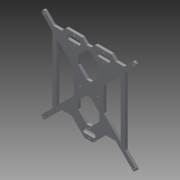
# Autodesk Inventor part: platform_redrawn
Saved by Autodesk Inventor 2015 (Build 190159000, 159)
## iProperties
Created: 2015-04-29
Part Number: platform_redrawn
Material: Generic
Document SubType Name: Modeling
Designer: X
Density: 1 g/cm^3
Appearance: Default
Author: X
Autodesk Inventor part; units mm, degrees
ref_plane "YZ Plane" through (0, 0, 0) normal (1, 0, 0) x (0, 1, 0)
ref_plane "XZ Plane" through (0, 0, 0) normal (0, 1, 0) x (-1, 0, 0)
ref_plane "XY Plane" through (0, 0, 0) normal (0, 0, 1) x (1, 0, 0)
sketch "Sketch1" plane through (0, 0, 0) normal (0, 1, 0) x (-1, 0, 0)
  line L0 (110, 110) -> (-110, 110)
  line L1 (-110, 110) -> (-110, -110)
  line L2 (-110, -110) -> (110, -110)
  line L3 (110, -110) -> (110, 110)
  line L4 (110, 110) -> (-110, -110) construction
  line L5 (-110, 110) -> (110, -110) construction
  point P0 (0, 0)
  dimension "d0" = 220
  dimension "d1" = 220
  constraints: 12 end point, 2 midpoint, 2 parallel, 1 horizontal, 1 perpendicular
  measures "d0" distance of L2.end L0.start
  measures "d1" distance of L0.start L0.end
extrude "Extrusion1" add sketch "Sketch1" along normal blind 6
sketch "Sketch2" plane through (0, 6, 0) normal (0, 1, 0) x (1, 0, 0)
  line L0 (110, 110) -> (-110, 110) construction
  line L1 (0, 110) -> (0, -110) construction
  line L2 (-110, 110) -> (-110, -110) projected
  line L3 (-110, 103) -> (-110, -103)
  line L4 (-110, -103) -> (-85, -78)
  line L5 (-85, -78) -> (-85, 78)
  line L6 (-85, 78) -> (-110, 103)
  line L7 (-75, 68) -> (-75, -68)
  line L8 (-75, -68) -> (-35, -28)
  line L9 (-35, -28) -> (-35, 28)
  line L10 (-35, 28) -> (-75, 68)
  line L11 (-110, -110) -> (110, -110) projected
  line L12 (-103, -110) -> (-83, -90)
  line L13 (-83, -90) -> (-63, -90)
  line L14 (-63, -90) -> (-43, -110)
  line L15 (-103, -110) -> (-43, -110)
  line L16 (-53, -100) -> (-15, -100)
  line L17 (-15, -100) -> (-15, -110)
  line L18 (-15, -110) -> (-53, -110)
  line L19 (-53, -110) -> (-53, -100)
  line L20 (-25, -110) -> (-5, -90)
  line L21 (-5, -90) -> (0, -90)
  line L22 (0, -80) -> (-5, -80)
  line L23 (-5, -80) -> (-25, -60)
  line L24 (-25, -60) -> (-25, -40)
  line L25 (-25, -40) -> (-5, -20)
  line L26 (-5, -20) -> (0, -20)
  line L27 (-103, 110) -> (-63, 70)
  line L28 (-63, 70) -> (-40, 70)
  line L29 (-40, 70) -> (0, 110)
  line L30 (0, 110) -> (-103, 110)
  line L31 (-10, 100) -> (0, 100)
  line L32 (0, 100) -> (0, 110)
  line L33 (0, 110) -> (-10, 110)
  line L34 (-10, 110) -> (-10, 100)
  line L35 (0, 70) -> (-5, 70)
  line L36 (-5, 70) -> (-25, 50)
  line L37 (-25, 50) -> (-25, 32)
  line L38 (-25, 32) -> (-5, 12)
  line L39 (-5, 12) -> (0, 12)
  line L40 (-110, 110) -> (110, 110) construction
  line L41 (110, 110) -> (110, -110)
  line L42 (110, 103) -> (110, -103)
  line L43 (110, -103) -> (85, -78)
  line L44 (85, -78) -> (85, 78)
  line L45 (85, 78) -> (110, 103)
  line L46 (75, 68) -> (75, -68)
  line L47 (75, -68) -> (35, -28)
  line L48 (35, -28) -> (35, 28)
  line L49 (35, 28) -> (75, 68)
  line L50 (110, -110) -> (-110, -110)
  line L51 (103, -110) -> (83, -90)
  line L52 (83, -90) -> (63, -90)
  line L53 (63, -90) -> (43, -110)
  line L54 (103, -110) -> (43, -110)
  line L55 (53, -100) -> (15, -100)
  line L56 (15, -100) -> (15, -110)
  line L57 (15, -110) -> (53, -110)
  line L58 (53, -110) -> (53, -100)
  line L59 (25, -110) -> (5, -90)
  line L60 (5, -90) -> (0, -90)
  line L61 (0, -80) -> (5, -80)
  line L62 (5, -80) -> (25, -60)
  line L63 (25, -60) -> (25, -40)
  line L64 (25, -40) -> (5, -20)
  line L65 (5, -20) -> (0, -20)
  line L66 (103, 110) -> (63, 70)
  line L67 (63, 70) -> (40, 70)
  line L68 (40, 70) -> (0, 110)
  line L69 (0, 110) -> (103, 110)
  line L70 (10, 100) -> (0, 100)
  line L71 (0, 110) -> (10, 110)
  line L72 (10, 110) -> (10, 100)
  line L73 (0, 70) -> (5, 70)
  line L74 (5, 70) -> (25, 50)
  line L75 (25, 50) -> (25, 32)
  line L76 (25, 32) -> (5, 12)
  line L77 (5, 12) -> (0, 12)
  line L78 (-15, -110) -> (0, -110)
  line L79 (110, -110) -> (-110, -110)
  line L80 (-110, -110) -> (110, -110)
  line L81 (15, -110) -> (0, -110)
  point P0 (0, 0)
  dimension "d4" = 206
  dimension "d6" = 25
  dimension "d7" = 135
  dimension "d8" = 7
  dimension "d10" = 10
  dimension "d11" = 40
  dimension "d12" = 135
  dimension "d13" = 7
  dimension "d14" = 20
  dimension "d15" = 135
  dimension "d16" = 38
  dimension "d17" = 10
  dimension "d20" = 25
  dimension "d21" = 60
  dimension "d22" = 10
  dimension "d23" = 135
  dimension "d24" = 57
  dimension "d25" = 7
  dimension "d26" = 40
  dimension "d27" = 10
  dimension "d28" = 30
  constraints: 158 end point, 39 symmetric about line, 21 point on line, 12 parallel, 7 collinear, 7 equal length, 7 perpendicular, 6 midpoint, 5 horizontal, 2 vertical
  measures "d4" distance of L3.end L3.start
  measures "d6" distance between parallel lines of L5 L3
  measures "d7" angle of L5 L6
  measures "d8" distance from line of L0 L3.start
  measures "d10" distance between parallel lines of L7 L5
  measures "d11" distance between parallel lines of L7 L9
  measures "d12" angle of L5 L4
  measures "d13" distance from line of L12.start L2
  measures "d14" distance between parallel lines of L11 L13
  measures "d15" angle of L14 L13
  measures "d16" distance of L16.start L16.end
  measures "d17" distance between parallel lines of L16 L13
  measures "d20" distance between parallel lines of L1 L24
  measures "d21" distance between parallel lines of L22 L26
  measures "d22" distance between parallel lines of L21 L22
  measures "d23" angle of L23 L24
  measures "d24" distance between parallel lines of L2 L19
  measures "d25" distance from line of L2 L27.start
  measures "d26" distance between parallel lines of L0 L28
  measures "d27" distance between parallel lines of L0 L31
  measures "d28" distance between parallel lines of L35 L31
extrude "Extrusion2" cut sketch "Sketch2" against normal through all
chamfer "Chamfer3" distance 3 angle 45 1 edges at (-110, 3, 110) measured on face at (-109.5, 3, 110)
chamfer "Chamfer4" distance 3 angle 45 1 edges at (110, 3, 110) measured on face at (110, 3, 109.5)
chamfer "Chamfer5" distance 3 angle 45 1 edges at (110, 3, -110) measured on face at (109.5, 3, -110)
chamfer "Chamfer6" distance 3 angle 45 1 edges at (-110, 3, -110) measured on face at (-109.5, 3, -110)
sketch "Sketch3" plane through (0, 6, 0) normal (0, 1, 0) x (1, 0, 0)
  line L0 (-10, 100) -> (10, 100) construction
  line L1 (0, 100) -> (0, -90) construction
  line L2 (5, -90) -> (-5, -90) construction
  line L3 (-11.5, 80) -> (11.5, 80)
  line L4 (15.5, 84) -> (15.5, 86)
  line L5 (11.5, 90) -> (-11.5, 90)
  line L6 (-15.5, 86) -> (-15.5, 84)
  line L7 (-15.5, 80) -> (15.5, 90) construction
  line L8 (15.5, 80) -> (-15.5, 90) construction
  line L9 (-53, -100) -> (-15, -100) projected
  arc A0 (-11.5, 90) -> (-15.5, 86) centre (-11.5, 86) ccw
  arc A1 (-15.5, 84) -> (-11.5, 80) centre (-11.5, 84) ccw
  arc A2 (15.5, 86) -> (11.5, 90) centre (11.5, 86) ccw
  arc A3 (11.5, 80) -> (15.5, 84) centre (11.5, 84) ccw
  line L10 (-46, -90) -> (-23, -90)
  line L11 (-19, -86) -> (-19, -84)
  line L12 (-23, -80) -> (-46, -80)
  line L13 (-50, -84) -> (-50, -86)
  line L14 (-50, -90) -> (-19, -80) construction
  line L15 (-19, -90) -> (-50, -80) construction
  arc A4 (-46, -80) -> (-50, -84) centre (-46, -84) ccw
  arc A5 (-50, -86) -> (-46, -90) centre (-46, -86) ccw
  arc A6 (-19, -84) -> (-23, -80) centre (-23, -84) ccw
  arc A7 (-23, -90) -> (-19, -86) centre (-23, -86) ccw
  line L16 (46, -90) -> (23, -90)
  line L17 (19, -86) -> (19, -84)
  line L18 (23, -80) -> (46, -80)
  line L19 (50, -84) -> (50, -86)
  arc A8 (50, -84) -> (46, -80) centre (46, -84) ccw
  arc A9 (46, -90) -> (50, -86) centre (46, -86) ccw
  arc A10 (23, -80) -> (19, -84) centre (23, -84) ccw
  arc A11 (19, -86) -> (23, -90) centre (23, -86) ccw
  point P0 (0, 0)
  point P1 (0, 85)
  point P2 (-34.5, -85)
  dimension "d50" = 10
  dimension "d51" = 31
  dimension "d52" = 10
  dimension "d56" = 4
  dimension "d57" = 4
  dimension "d58" = 10
  dimension "d60" = 14
  constraints: 34 end point, 24 point on circle, 17 point on line, 16 tangent, 12 centre point, 12 symmetric about line, 6 equal radius, 6 midpoint, 6 parallel, 2 horizontal, 2 perpendicular, 4 other
  measures "d50" distance between parallel lines of L0 L5
  measures "d51" distance of L7.start L8.start
  measures "d52" distance of L8.start L7.end
  measures "d56" radius of A0
  measures "d57" radius of A4
  measures "d58" distance between parallel lines of L9 L10
  measures "d60" distance from line of L2.end L11
extrude "Extrusion3" cut sketch "Sketch3" against normal through all
sketch "Sketch4" plane through (0, 6, 0) normal (0, 1, 0) x (1, 0, 0)
  line L0 (-10, 100) -> (10, 100) construction
  line L1 (0, 100) -> (0, -90) construction
  line L2 (5, -90) -> (-5, -90) construction
  line L3 (-63, 70) -> (-103, 110) projected
  line L4 (-5, 70) -> (5, 70) projected
  line L5 (-46, -80) -> (-23, -80) projected
  line L6 (-23, -90) -> (-46, -90) projected
  line L7 (-34.5, -75) -> (-34.5, -95) construction
  line L8 (-5, -20) -> (5, -20) construction
  line L9 (-110, 107) -> (-107, 110) construction
  line L10 (-107, -110) -> (-110, -107) construction
  line L11 (-103, -110) -> (-83, -90) construction
  point P0 (0, 0)
  point P1 (0, 95)
  point P2 (0, 75)
  point P3 (-104.546, 104.475)
  point P4 (-104.546, -104.475)
  point P5 (-20.49, 0.037)
  point P6 (104.546, 104.475)
  point P7 (104.546, -104.475)
  point P8 (34.5, -75)
  point P9 (34.5, -95)
  point P10 (20.49, 0.037)
  dimension "d63" = 5
  dimension "d64" = 5
  dimension "d65" = 5
  dimension "d66" = 5
  dimension "d67" = 5
  dimension "d68" = 11.5
  dimension "d69" = 20.49
  dimension "d70" = 20.037
  dimension "d71" = 5.642
  dimension "d72" = 5.642
  dimension "d73" = 5
  constraints: 5 symmetric about line, 4 end point, 2 midpoint, 2 point on line, 1 perpendicular
  measures "d63" distance from line of L3 point (-104.546, 104.475)
  measures "d64" distance from line of L0 point (0, 95)
  measures "d65" distance from line of point (0, 75) L4
  measures "d66" distance from line of L7.start L5
  measures "d67" distance from line of L7.end L6
  measures "d68" horizontal distance of L7.start L5.end
  measures "d69" distance from line of L1 point (-20.49, 0.037)
  measures "d70" distance from line of L8 point (-20.49, 0.037)
  measures "d71" distance from line of L9 point (-104.546, 104.475)
  measures "d72" distance from line of L10 point (-104.546, -104.475)
  measures "d73" distance from line of L11 point (-104.546, -104.475)
hole "Hole1" at (0, 6, -95) at (0, 6, -75) at (-104.546, 6, -104.475) at (-104.546, 6, 104.475) at (-34.5, 6, 75) at (-34.5, 6, 95) at (-20.49, 6, -0.037) at (104.546, 6, -104.475) at (20.49, 6, -0.037) at (34.5, 6, 75) at (34.5, 6, 95) at (104.546, 6, 104.475) direction (0, -1, 0) diameter 3.6 end through all
body "Solid1"
